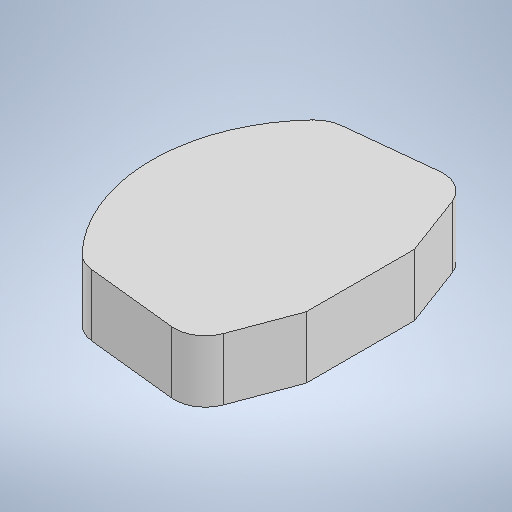
# Autodesk Inventor part: tuningpeg
Saved by Autodesk Inventor 2025.2 (Build 292293000, 293)
## iProperties
Created: 2025-04-17
Part Number: tuningpeg
Material: Generic
Document SubType Name: Modeling
Designer: 3lin2
Density: 1 g/cm^3
Appearance: Default
Author: 3lin2
Autodesk Inventor part; units mm, degrees
ref_plane "YZ Plane" through (0, 0, 0) normal (1, 0, 0) x (0, 1, 0)
ref_plane "XZ Plane" through (0, 0, 0) normal (0, 1, 0) x (-1, 0, 0)
ref_plane "XY Plane" through (0, 0, 0) normal (0, 0, 1) x (1, 0, 0)
sketch "Sketch1" plane through (0, 0, 0) normal (0, 1, 0) x (-1, 0, 0)
  line L0 (0, 3.5) -> (0, -3.5)
  line L1 (0, -3.5) -> (2, -8.85)
  line L2 (0, 3.5) -> (2, 8.85)
  line L3 (2, 8.85) -> (10, 8)
  line L4 (2, -8.85) -> (10, -8)
  arc A0 (10, -8) -> (10, 8) centre (2.6071, 0) ccw
  point P0 (0, 0)
  point P1 (0, 0)
  point P2 (13.5, 0)
  dimension "d0" = 7
  dimension "d1" = 3.5
  dimension "d2" = 5.35
  dimension "d3" = 2
  dimension "d4" = 5.35
  dimension "d5" = 2
  dimension "d6" = 8
  dimension "d7" = 8
  dimension "d8" = 4.5
  dimension "d9" = 4.5
  dimension "d10" = 13.5
  constraints: 10 end point, 3 point on circle, 1 centre point, 1 midpoint, 1 vertical
  measures "d0" distance of L0.start L0.end
  measures "d1" distance of L0.end point (0, 0)
  measures "d2" vertical distance of L1.end L0.end
  measures "d3" horizontal distance of L0.end L1.end
  measures "d4" vertical distance of L2.end L0.start
  measures "d5" horizontal distance of L0.start L2.end
  measures "d6" horizontal distance of L3.end L2.end
  measures "d7" horizontal distance of L1.end L4.end
  measures "d8" vertical distance of L0.start L3.end
  measures "d9" vertical distance of L4.end L0.end
  measures "d10" distance of point (0, 0) point (13.5, 0)
extrude "Extrusion1" add sketch "Sketch1" along normal blind 4
fillet "Fillet1" radius 2 4 edges at (-2, 2, -8.85) (-2, 2, 8.85) (-10, 2, 8) (-10, 2, -8)
body "Solid1"
